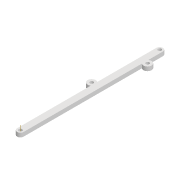
# Autodesk Inventor part: Part_3
Saved by Autodesk Inventor 2022 (Build 260153000, 153)
## iProperties
Created: 2022-04-22
Part Number: Part_3
Material: Generic
Document SubType Name: Modeling
Designer: dell
Density: 1 g/cm^3
Appearance: Default
Mass: 7.44781 g
Surface Area: 52.1011 cm^2
Volume: 7.44781 cm^3
Author: dell
Autodesk Inventor part; units mm, degrees
ref_plane "YZ Plane" through (0, 0, 0) normal (1, 0, 0) x (0, 1, 0)
ref_plane "XZ Plane" through (0, 0, 0) normal (0, 1, 0) x (-1, 0, 0)
ref_plane "XY Plane" through (0, 0, 0) normal (0, 0, 1) x (1, 0, 0)
sketch "Sketch1" plane through (0, 0, 0) normal (0, 1, 0) x (-1, 0, 0)
  line L0 (0, 0) -> (0, -172) construction
  line L1 (4, 0) -> (4, -172)
  line L2 (-4, -172) -> (-4, 0)
  arc A0 (4, 0) -> (-4, 0) centre (0, 0) ccw
  arc A1 (-4, -172) -> (4, -172) centre (0, -172) ccw
  circle A2 centre (0, 0) radius 2.1
  circle A3 centre (0, -172) radius 2.1
  circle A4 centre (7, -93) radius 2.1
  circle A5 centre (7, -93) radius 5
  circle A6 centre (-7, -150) radius 2.1
  circle A7 centre (-7, -150) radius 5
  point P0 (0, -86)
  point P1 (4, -89)
  point P2 (4, -99.3597)
  point P3 (4, -100.6403)
  point P4 (4, -97)
  point P5 (-4, -146)
  point P6 (-4, -154)
  dimension "d0" = 172
  dimension "d1" = 8
  dimension "d2" = 4.2
  dimension "d3" = 4.2
  dimension "d8" = 4.2
  dimension "d9" = 93
  dimension "d10" = 3
  dimension "d11" = 10
  dimension "d12" = 4.2
  dimension "d13" = 10
  dimension "d15" = 3
  dimension "d16" = 150
  constraints: 8 centre point, 8 end point, 4 coincident, 4 point on circle, 4 tangent, 1 midpoint, 1 parallel, 1 vertical
  measures "d0" distance of L0.end L0.start
  measures "d1" distance between parallel lines of L2 L1
  measures "d2" diameter of A2
  measures "d3" diameter of A3
  measures "d8" diameter of A4
  measures "d9" vertical distance of L0.start A4.centre
  measures "d10" distance from line of L1 A4.centre
  measures "d11" diameter of A5
  measures "d12" diameter of A6
  measures "d13" diameter of A7
  measures "d15" distance from line of L2 A6.centre
  measures "d16" vertical distance of L0.start A6.centre
extrude "Extrusion1" add sketch "Sketch1" along normal blind 5
body "Solid1"
